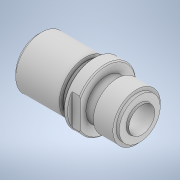
# Autodesk Inventor part: 411. Штуцер гибкого вала
Saved by Autodesk Inventor 2021 (Build 250183000, 183)
## iProperties
Created: 2021-04-18
Part Number: 411. Штуцер гибкого вала
Material: Типовые
Document SubType Name: Modeling
Designer: Данил
Density: 1 g/cm^3
Appearance: По умолчанию
Author: Данил
Autodesk Inventor part; units mm, degrees
ref_plane "YZ Plane" through (0, 0, 0) normal (1, 0, 0) x (0, 1, 0)
ref_plane "XZ Plane" through (0, 0, 0) normal (0, 1, 0) x (-1, 0, 0)
ref_plane "XY Plane" through (0, 0, 0) normal (0, 0, 1) x (1, 0, 0)
sketch "Эскиз1" plane through (0, 0, 0) normal (0, 0, 1) x (1, 0, 0)
  line L0 (-24, 0) -> (24, 0)
  line L1 (0, -5.5) -> (-23.2, -5.5)
  line L2 (-24, -6.3) -> (-24, -10.4)
  line L3 (0, -5.5) -> (0, -6)
  line L4 (0, -6) -> (24, -6)
  line L5 (-23.2, -5.5) -> (-24, -6.3)
  line L6 (-22.4, -12) -> (-2.2, -12)
  line L7 (-22.4, -12) -> (-24, -10.4)
  line L8 (-1.4, -11.2) -> (-1.4, -11)
  line L9 (-1.4, -11) -> (1.6, -11)
  line L10 (-2.2, -12) -> (-1.4, -11.2)
  line L11 (1.6, -11) -> (1.6, -13.5)
  line L12 (2.1, -14) -> (7.1, -14)
  line L13 (7.6, -13.5) -> (7.6, -9.5)
  line L14 (7.6, -9.5) -> (12.6, -9.5)
  line L15 (2.1, -14) -> (1.6, -13.5)
  line L16 (7.1, -14) -> (7.6, -13.5)
  line L17 (12.6, -9.5) -> (12.6, -11)
  line L18 (12.6, -11) -> (21.6, -11)
  line L19 (21.6, -11) -> (21.6, -9.5)
  line L20 (24, -6) -> (23, -6.2309)
  line L21 (23, -6.2309) -> (23, -9.5)
  line L22 (23, -9.5) -> (21.6, -9.5)
  point P0 (0, 0)
  point P1 (0, 0)
  point P2 (-24, -5.5)
  point P3 (-24, -12)
  point P4 (-1.4, -12)
  point P5 (1.6, -14)
  point P6 (7.6, -14)
  dimension "d0" = 48
  dimension "d24" = 12
  dimension "d25" = 11
  dimension "d26" = 24
  dimension "d27" = 0.8
  dimension "d28" = 45
  dimension "d29" = 24
  dimension "d30" = 1.6
  dimension "d31" = 45
  dimension "d32" = 22
  dimension "d33" = 0.8
  dimension "d34" = 45
  dimension "d35" = 3
  dimension "d36" = 24
  dimension "d37" = 0.5
  dimension "d38" = 45
  dimension "d39" = 0.5
  dimension "d40" = 45
  dimension "d41" = 19
  dimension "d42" = 6
  dimension "d43" = 5
  dimension "d44" = 22
  dimension "d47" = 13
  dimension "d49" = 14
  dimension "d50" = 19
  dimension "d51" = 1
  dimension "d52" = 28
  constraints: 46 end point, 10 point on line, 9 perpendicular, 5 vertical, 3 horizontal, 2 vertical alignment, 1 coincident, 1 midpoint
  measures "d0" distance of L0.start L0.end
  measures "d24" diameter of L4 L0
  measures "d25" diameter of L1 L0
  measures "d26" distance of L1.start point (-24, -5.5)
  measures "d27" distance of L1.end point (-24, -5.5)
  measures "d28" angle of L1 L5
  measures "d29" diameter of L6 L0
  measures "d30" distance of L6.start point (-24, -12)
  measures "d31" angle of L6 L7
  measures "d32" diameter of L9 L0
  measures "d33" distance of L6.end point (-1.4, -12)
  measures "d34" angle of L6 L10
  measures "d35" distance of L8.end L9.end
  measures "d36" horizontal distance of L9.end L6.start
  measures "d37" distance of L12.start point (1.6, -14)
  measures "d38" angle of L12 L15
  measures "d39" distance of L12.end point (7.6, -14)
  measures "d40" angle of L12 L16
  measures "d41" diameter of L14 L0
  measures "d42" distance between parallel lines of L11 L13
  measures "d43" distance of L13.end L14.end
  measures "d44" diameter of L18 L0
  measures "d47" angle of L0 L20
  measures "d49" distance between parallel lines of L13 L19
  measures "d50" diameter of L22 L0
  measures "d51" distance from line of L4.end L21
  measures "d52" diameter of L12 L0
revolve "Вращение1" add sketch "Эскиз1" angle 360 about axis through (-24, 0, 0) along (1, 0, 0)
sketch "Эскиз2" plane through (0, 0, 0) normal (0, 1, 0) x (-1, 0, 0)
  line L0 (-1.6, -13.5) -> (-1.6, 13.5) projected
  line L1 (-7.1, 14) -> (-2.1, 14) projected
  line L2 (-7.6, 13.5) -> (-7.1, 14) projected
  line L3 (-7.6, -13.5) -> (-7.6, 13.5) projected
  line L4 (-2.1, 14) -> (-1.6, 13.5) projected
  line L5 (-3.6, 14) -> (-3.6, 12)
  line L6 (-3.6, 12) -> (-7.6, 12)
  line L7 (2.2, 12) -> (22.4, 12) projected
  point P0 (0, 0)
  dimension "d54" = 2
  constraints: 4 end point, 2 point on line, 1 collinear, 1 perpendicular, 1 vertical
  measures "d54" distance between parallel lines of L5 L0
extrude "Выдавливание1" cut sketch "Эскиз2" along normal through all both and the other way through all
fillet "Сопряжение1" radius 0.3 1 edges at (3.6, 0, 12)
equation "\"d39\" = d37"
equation "\"d40\" = d38"
